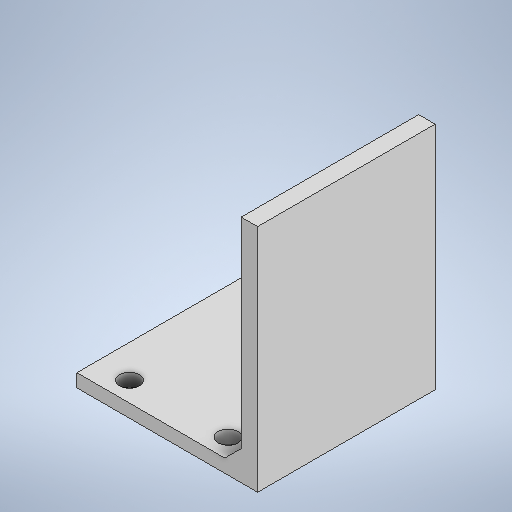
# Autodesk Inventor part: obudowa_łoż_pion_1
Saved by Autodesk Inventor 2025 (Build 290162000, 162)
## iProperties
Created: 2024-04-14
Part Number: obudowa_łoż_pion_1
Material: Ogólny
Document SubType Name: Modeling
Designer: user
Density: 1 g/cm^3
Appearance: Domyślna
Author: user
Autodesk Inventor part; units mm, degrees
ref_plane "YZ Plane" through (0, 0, 0) normal (1, 0, 0) x (0, 1, 0)
ref_plane "XZ Plane" through (0, 0, 0) normal (0, 1, 0) x (-1, 0, 0)
ref_plane "XY Plane" through (0, 0, 0) normal (0, 0, 1) x (1, 0, 0)
sketch "Szkic1" plane through (0, 0, 0) normal (0, 1, 0) x (-1, 0, 0)
  line L0 (25, 27) -> (-25, 27)
  line L1 (-25, 27) -> (-25, -27)
  line L2 (-25, -27) -> (25, -27)
  line L3 (25, -27) -> (25, 27)
  line L4 (-25, 27) -> (25, -27) construction
  circle A0 centre (15, 21) radius 3
  line L5 (25, 0) -> (-25, 0)
  line L6 (0, 27) -> (0, -27)
  circle A1 centre (15, -21) radius 3
  circle A2 centre (-15, 21) radius 3
  circle A3 centre (-15, -21) radius 3
  line L7 (-25, 27) -> (-30, 27)
  line L8 (-30, 27) -> (-30, -27)
  line L9 (-30, -27) -> (-25, -27)
  line L10 (-25, -27) -> (-25, 27)
  point P0 (0, 0)
  point P1 (-27.5, 27)
  point P2 (-25, -27)
  dimension "d0" = 50
  dimension "d5" = 10
  dimension "d7" = 6
  dimension "d8" = 6
  dimension "d9" = 5
  dimension "d10" = 54
  dimension "d12" = 54
  constraints: 22 end point, 6 midpoint, 4 centre point, 4 parallel, 3 symmetric about line, 2 horizontal, 2 perpendicular, 3 other
  measures "d0" distance of L2.end L1.end
  measures "d5" distance from line of A0.centre L3
  measures "d7" distance from line of A0.centre L0
  measures "d8" diameter of A0
  measures "d9" distance between parallel lines of L1 L8
  measures "d10" distance from line of point (-27.5, 27) L9
  measures "d12" distance between parallel lines of L2 L0
sketch "Szkic2" plane through (0, 0, 0) normal (0, 1, 0) x (-1, 0, 0)
  point P0 (0, 0)
extrude "Wyciągnięcie proste1" add sketch "Szkic1" along normal blind 4 contours L3 L5 L6 L0 | L6 L5 L1 L0 | L3 L2 L6 L5 | L6 L2 L1 L5
extrude "Wyciągnięcie proste2" add sketch "Szkic1" along normal blind 70 contours L1 L9 L8 L7
sketch "Szkic3" plane through (-25, 0, 27) normal (0, 0, 1) x (1, 0, 0)
  line L0 (50, 4) -> (50, 70) projected
  line L1 (50, 9) -> (45, 4)
  line L2 (0, 4) -> (50, 4) projected
  line L3 (50, 9) -> (57.0711, 9) construction
  point P0 (25, 0)
  dimension "d17" = 135
  dimension "d18" = 5
  constraints: 4 end point, 2 point on line, 1 equal length, 1 horizontal
  measures "d17" angle of L1 L3
  measures "d18" horizontal distance of L1.start L1.end
extrude "Wyciągnięcie proste3" add sketch "Szkic3" against normal blind 54
sketch "Szkic4" plane through (0, 4, 0) normal (0, 1, 0) x (1, 0, 0)
  point P0 (0, 0)
